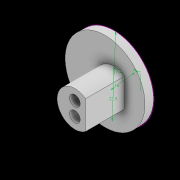
# Autodesk Inventor part: Part8
Saved by Autodesk Inventor 2022.2 (Build 262287010, 287A)
## iProperties
Created: 2022-06-02
Part Number: Part8
Material: Generic
Document SubType Name: Modeling
Designer: Árni Þór Þorgeirsson
Density: 1 g/cm^3
Appearance: Default
Author: Árni Þór Þorgeirsson
Autodesk Inventor part; units mm, degrees
ref_plane "YZ Plane" through (0, 0, 0) normal (1, 0, 0) x (0, 1, 0)
ref_plane "XZ Plane" through (0, 0, 0) normal (0, 1, 0) x (-1, 0, 0)
sketch "Sketch1" plane through (0, 0, 0) normal (0, 0, 1) x (1, 0, 0)
  circle A0 centre (0, 0) radius 11.25
  line L0 (0, 0) -> (2.5, 0)
  circle A1 centre (2.5, 0) radius 5
  line L1 (5.5, 6.7455) -> (5.5, -7.7933)
  point P0 (7.5, 0)
  point P1 (7.5, 0)
  point P2 (5.5, -4)
  point P3 (5.5, 4)
  dimension "d2" = 10
  dimension "d0" = 22.5
  dimension "d1" = 2.5
  dimension "d3" = 2
  constraints: 4 end point, 3 coincident, 1 centre point, 1 horizontal, 1 vertical, 3 other
  measures "d0" diameter of A0
  measures "d1" distance of L0.start L0.end
  measures "d3" distance from line of point (7.5, 0) L1
extrude "Extrusion1" add sketch "Sketch1" along normal blind 2.5 contours A0 | A1 L1 | L1 A1
extrude "Extrusion2" add sketch "Sketch1" along normal blind 11 from surface at 2.5 contours L1 A1 picked at (2.8333, 0)
sketch "Sketch2" plane through (2.5, 0, 13.5) normal (0, 0, 1) x (1, 0, 0)
  line L0 (0, 0) -> (0, 2)
  line L1 (0, 0) -> (0, -1.8526)
  line L2 (0, -1.8526) -> (2, -1.8526)
  point P0 (-2.5, 0)
  dimension "d8" = 2
  dimension "d9" = 2
  constraints: 6 end point, 1 perpendicular, 1 vertical
  measures "d8" distance of L0.start L0.end
  measures "d9" distance of L1.end L2.end
hole "Hole1" at (2.5, 2, 13.5) at (2.5, -1.8526, 13.5) direction (0, 0, -1) diameter 3 depth 4
draft "FaceDraft1" angle 2.5 pull direction (0, 0, -1) faces at (11.1043, -1.8046, 1.6667) fixed edges at (-11.25, 0, 2.5)
sketch "Sketch3" plane through (0, 0, 20) normal (0, 0, 1) x (1, 0, 0)
  arc A0 (5.5, 4) -> (5.5, -4) centre (2.5, 0) ccw projected
  circle A1 centre (2.5, 2) radius 1.5 projected
  circle A2 centre (2.5, -1.8526) radius 1.5 projected
  line L0 (2.5, 5) -> (27.5, 5)
  line L1 (2.5, -5) -> (27.5, -5)
  line L2 (27.5, -5) -> (27.5, 5)
  point P0 (0, 0)
  dimension "d18" = 25
  dimension "d19" = 25
  constraints: 6 end point, 2 horizontal, 2 point on circle, 1 perpendicular
  measures "d18" distance of L0.start L0.end
  measures "d19" distance of L1.start L1.end
body "Solid1"
